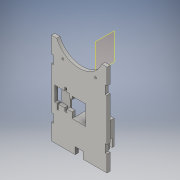
# Autodesk Inventor part: Backhalf
Saved by Autodesk Inventor 2016 (Build 200138000, 138)
## iProperties
Created: 2017-03-04
Part Number: Backhalf
Material: Generic
Document SubType Name: Modeling
Designer: Owner
Density: 1 g/cm^3
Appearance: Default
Author: Owner
Autodesk Inventor part; units mm, degrees
ref_plane "YZ Plane" through (0, 0, 0) normal (1, 0, 0) x (0, 1, 0)
ref_plane "XZ Plane" through (0, 0, 0) normal (0, 1, 0) x (-1, 0, 0)
ref_plane "XY Plane" through (0, 0, 0) normal (0, 0, 1) x (1, 0, 0)
sketch "Sketch1" plane through (0, 0, 0) normal (0, 0, 1) x (1, 0, 0)
  line L0 (31.75, -57.15) -> (31.75, 82.55)
  line L1 (31.75, 82.55) -> (-44.45, 82.55)
  line L2 (-44.45, 82.55) -> (-44.45, -57.15)
  arc A0 (-44.45, -57.15) -> (31.75, -57.15) centre (-6.35, -57.15) ccw
  line L3 (31.75, -57.15) -> (31.75, -209.55)
  line L4 (31.75, -209.55) -> (-44.45, -209.55)
  line L5 (-44.45, -209.55) -> (-44.45, -57.15)
  line L6 (31.75, -57.15) -> (-44.45, -57.15)
  circle A1 centre (-6.35, -57.15) radius 38.1
  point P0 (0, 0)
  dimension "d0" = 152.4
  dimension "d6" = 76.2
  constraints: 14 end point, 3 perpendicular, 2 centre point, 2 point on circle, 2 tangent, 1 coincident, 1 concentric, 1 vertical
  measures "d0" distance of L0.start L3.end
  measures "d6" distance of L3.end L4.end
extrude "Extrusion1" add sketch "Sketch1" against normal blind 5 contours L3 L4 L5 A0
sketch "Sketch2" plane through (0, 0, 0) normal (0, 0, 1) x (1, 0, 0)
  arc A0 (-44.45, -57.15) -> (31.75, -57.15) centre (-6.35, -57.15) ccw projected
  line L0 (31.75, -57.15) -> (31.75, -209.55) projected
  line L1 (-44.45, -57.15) -> (31.75, -57.15)
  line L2 (31.75, -57.15) -> (31.75, -72.15)
  line L3 (31.75, -72.15) -> (-44.45, -72.15)
  line L4 (-44.45, -72.15) -> (-44.45, -57.15)
  point P0 (0, 0)
  dimension "d3" = 15
  constraints: 8 end point, 2 parallel, 1 horizontal, 1 perpendicular, 1 point on line
  measures "d3" distance of L3.end L1.start
extrude "Extrusion2" cut sketch "Sketch2" against normal blind 5 contours L1 A0 L3 | A0 L3 L4 | L0 L3 A0
sketch "Sketch3" plane through (0, 0, -5) normal (0, 0, -1) x (-1, 0, 0)
  line L0 (16.51, -146.85) -> (16.51, -159.55) projected
  line L1 (-3.81, -159.55) -> (-3.81, -146.85) projected
  line L2 (16.51, -159.55) -> (16.51, -161.55)
  line L3 (-3.81, -146.85) -> (-3.81, -144.85)
  line L4 (4.857, -150.5555) -> (16.51, -161.55)
  line L5 (8.3369, -156.3105) -> (-3.81, -144.85)
  line L6 (16.51, -141.135) -> (12.446, -141.135)
  line L7 (16.51, -165.265) -> (12.446, -165.265)
  line L8 (16.51, -141.135) -> (17.51, -141.135)
  line L9 (17.51, -141.135) -> (17.51, -138.135)
  line L10 (17.51, -138.135) -> (-3.81, -138.135)
  line L11 (-3.81, -138.135) -> (-3.81, -163.265)
  line L12 (-3.81, -163.265) -> (-3.81, -164.265)
  line L13 (17.51, -138.135) -> (17.51, -165.265)
  line L14 (17.51, -165.265) -> (17.51, -168.265)
  line L15 (17.51, -168.265) -> (-3.81, -168.265)
  line L16 (-3.81, -168.265) -> (-3.81, -164.265)
  point P0 (0, 0)
  point P1 (17.51, -164.265)
  dimension "d7" = 2
  dimension "d8" = 2
  dimension "d28" = 1
  dimension "d29" = 3
  dimension "d30" = 1
  dimension "d73" = 3
  constraints: 30 end point, 5 perpendicular, 3 horizontal, 3 point on line, 3 vertical, 1 parallel, 4 other
  measures "d7" distance of L0.end L2.end
  measures "d8" distance of L1.end L3.end
  measures "d28" distance of L6.start L8.end
  measures "d29" distance of L8.end L9.end
  measures "d30" distance of L11.end L12.end
  measures "d73" distance of L13.end L14.end
extrude "Extrusion3" cut sketch "Sketch3" against normal blind 5
sketch "Sketch4" plane through (0, 0, -5) normal (0, 0, -1) x (-1, 0, 0)
  line L0 (-31.75, -72.15) -> (-28.673, -72.15) projected
  line L1 (-31.75, -72.15) -> (-36.75, -72.15)
  line L2 (-36.75, -72.15) -> (-36.75, -209.55)
  line L3 (-36.75, -209.55) -> (-36.75, -214.55)
  line L4 (-36.75, -214.55) -> (44.45, -214.55)
  line L5 (44.45, -214.55) -> (49.45, -214.55)
  line L6 (49.45, -214.55) -> (49.45, -72.15)
  line L7 (49.45, -72.15) -> (44.45, -72.15)
  line L8 (44.45, -72.15) -> (44.45, -214.55)
  line L9 (44.45, -214.55) -> (49.45, -214.55)
  line L10 (49.45, -214.55) -> (49.45, -72.15)
  line L11 (49.45, -214.55) -> (-36.75, -214.55)
  line L12 (-36.75, -214.55) -> (-36.75, -209.55)
  line L13 (-36.75, -209.55) -> (49.45, -209.55)
  line L14 (49.45, -209.55) -> (49.45, -214.55)
  line L15 (-36.75, -214.55) -> (-31.75, -214.55)
  line L16 (-31.75, -214.55) -> (-31.75, -72.15)
  line L17 (-31.75, -72.15) -> (-36.75, -72.15)
  line L18 (-36.75, -72.15) -> (-36.75, -214.55)
  point P0 (0, 0)
  dimension "d11" = 5
  dimension "d12" = 5
  dimension "d13" = 5
  constraints: 36 end point, 6 parallel, 6 perpendicular, 4 horizontal, 3 point on line
  measures "d11" distance of L0.start L1.end
  measures "d12" distance of L2.end L3.end
  measures "d13" distance of L4.end L5.end
extrude "Extrusion4" add sketch "Sketch4" against normal blind 5
sketch "Sketch6" plane through (-49.45, -214.55, 0) normal (0, -1, 0) x (1, 0, 0)
  line L0 (32.94, 0) -> (53.26, 0) projected
  line L1 (43.1, 0) -> (36.75, 0)
  line L2 (36.75, 0) -> (49.45, 0)
  line L3 (86.2, -5) -> (0, -5) projected
  line L4 (49.45, 0) -> (36.75, 0)
  line L5 (36.75, 0) -> (36.75, -5)
  line L6 (36.75, -5) -> (49.45, -5)
  line L7 (49.45, -5) -> (49.45, 0)
  point P0 (64.1616, -5)
  dimension "d18" = 6.35
  dimension "d19" = 12.7
  constraints: 12 end point, 2 parallel, 2 point on line, 1 collinear, 1 horizontal, 1 midpoint, 1 perpendicular
  measures "d18" distance of L1.start L1.end
  measures "d19" distance of L1.end L2.end
extrude "Extrusion6" add sketch "Sketch6" along normal blind 10.16
sketch "Sketch7" plane through (0, 0, -5) normal (0, 0, -1) x (-1, 0, 0)
  line L0 (12.7, -224.71) -> (0, -224.71) projected
  line L1 (6.35, -224.71) -> (6.35, -220.9)
  circle A0 centre (6.35, -220.9) radius 1.75
  point P0 (0, 0)
  dimension "d26" = 3.81
  dimension "d27" = 3.5
  constraints: 2 end point, 1 centre point, 1 coincident, 1 midpoint, 1 vertical
  measures "d26" distance of L1.start L1.end
  measures "d27" diameter of A0
extrude "Extrusion7" cut sketch "Sketch7" against normal blind 6.35
sketch "Sketch8" plane through (0, 0, -5) normal (0, 0, -1) x (-1, 0, 0)
  line L0 (44.45, -136.69) -> (28.448, -136.69) projected
  line L1 (44.45, -158.28) -> (44.45, -137.96) projected
  line L2 (44.45, -136.69) -> (44.45, -137.96) projected
  line L3 (44.45, -158.28) -> (44.45, -159.55) projected
  line L4 (44.45, -159.55) -> (28.448, -159.55) projected
  line L5 (39.116, -159.55) -> (40.132, -159.55) projected
  line L6 (39.116, -159.55) -> (39.116, -162.09) projected
  line L7 (40.132, -162.09) -> (39.116, -162.09) projected
  line L8 (40.132, -159.55) -> (40.132, -162.09) projected
  line L9 (25.908, -137.96) -> (21.59, -137.96) projected
  line L10 (21.59, -153.2) -> (21.59, -137.96) projected
  line L11 (21.59, -158.28) -> (21.59, -153.2) projected
  line L12 (25.908, -158.28) -> (21.59, -158.28) projected
  line L13 (25.908, -158.28) -> (25.908, -164.122) projected
  line L14 (25.908, -164.122) -> (28.448, -164.122) projected
  line L15 (28.448, -158.28) -> (28.448, -164.122) projected
  line L16 (44.45, -158.28) -> (28.448, -158.28) projected
  line L17 (44.45, -158.28) -> (44.45, -137.96) projected
  line L18 (44.45, -137.96) -> (28.448, -137.96) projected
  line L19 (28.448, -132.118) -> (28.448, -137.96) projected
  line L20 (25.908, -132.118) -> (28.448, -132.118) projected
  line L21 (25.908, -132.118) -> (25.908, -137.96) projected
  line L22 (25.908, -136.69) -> (21.59, -136.69) projected
  line L23 (21.59, -136.69) -> (21.59, -137.96) projected
  line L24 (25.908, -159.55) -> (21.59, -159.55) projected
  line L25 (21.59, -159.55) -> (16.51, -159.55)
  line L26 (21.59, -146.85) -> (16.51, -146.85)
  line L27 (17.51, -140.135) -> (17.51, -166.265) projected
  line L28 (44.45, -159.55) -> (21.59, -159.55)
  line L29 (21.59, -159.55) -> (21.59, -136.69)
  line L30 (21.59, -136.69) -> (44.45, -136.69)
  line L31 (44.45, -136.69) -> (44.45, -159.55)
  line L32 (28.448, -132.118) -> (25.908, -132.118)
  line L33 (25.908, -132.118) -> (25.908, -136.69)
  line L34 (25.908, -136.69) -> (28.448, -136.69)
  line L35 (28.448, -136.69) -> (28.448, -132.118)
  line L36 (25.908, -159.55) -> (28.448, -159.55)
  line L37 (28.448, -159.55) -> (28.448, -164.122)
  line L38 (28.448, -164.122) -> (25.908, -164.122)
  line L39 (25.908, -164.122) -> (25.908, -159.55)
  line L40 (40.132, -162.09) -> (39.116, -162.09)
  line L41 (39.116, -162.09) -> (39.116, -159.55)
  line L42 (39.116, -159.55) -> (40.132, -159.55)
  line L43 (40.132, -159.55) -> (40.132, -162.09)
  line L44 (16.51, -146.85) -> (21.59, -146.85)
  line L45 (21.59, -146.85) -> (21.59, -159.55)
  line L46 (21.59, -159.55) -> (16.51, -159.55)
  line L47 (16.51, -159.55) -> (16.51, -146.85)
  line L48 (40.132, -159.55) -> (40.64, -159.55)
  line L49 (40.64, -159.55) -> (40.64, -167.805)
  line L50 (40.64, -167.805) -> (39.116, -167.805)
  line L51 (39.116, -167.805) -> (38.608, -167.805)
  line L52 (38.608, -167.805) -> (38.608, -159.55)
  line L53 (40.64, -167.805) -> (38.608, -167.805)
  line L54 (38.608, -167.805) -> (38.608, -159.55)
  line L55 (38.608, -159.55) -> (40.64, -159.55)
  line L56 (40.64, -159.55) -> (40.64, -167.805)
  line L57 (28.448, -136.69) -> (28.948, -136.69)
  line L58 (28.948, -136.69) -> (28.948, -132.118)
  line L59 (28.948, -132.118) -> (28.948, -131.618)
  line L60 (28.948, -131.618) -> (25.908, -131.618)
  line L61 (25.908, -131.618) -> (25.408, -131.618)
  line L62 (25.408, -131.618) -> (25.408, -136.69)
  line L63 (44.45, -148.12) -> (42.0007, -148.12)
  line L64 (28.448, -164.122) -> (28.448, -158.28)
  line L65 (25.908, -164.122) -> (28.448, -164.122)
  line L66 (25.908, -164.122) -> (25.908, -158.28)
  line L67 (28.448, -164.122) -> (25.908, -164.122)
  line L68 (25.908, -164.122) -> (25.908, -159.55)
  line L69 (28.448, -159.55) -> (28.448, -164.122)
  line L70 (28.948, -159.55) -> (28.948, -164.122)
  line L71 (28.948, -164.122) -> (28.948, -164.622)
  line L72 (28.948, -164.622) -> (25.908, -164.622)
  line L73 (25.908, -164.622) -> (25.408, -164.622)
  line L74 (25.408, -164.622) -> (25.408, -159.55)
  line L75 (28.948, -159.55) -> (25.408, -159.55)
  line L76 (25.408, -159.55) -> (25.408, -164.622)
  line L77 (25.408, -164.622) -> (28.948, -164.622)
  line L78 (28.948, -164.622) -> (28.948, -159.55)
  point P0 (0, 0)
  dimension "d33" = 0.508
  dimension "d34" = 8.255
  dimension "d35" = 0.508
  dimension "d45" = 0.5
  dimension "d46" = 0.5
  dimension "d47" = 0.5
  constraints: 100 end point, 14 parallel, 12 perpendicular, 10 horizontal, 9 point on line, 9 symmetric about line, 1 midpoint, 1 vertical, 3 other
  measures "d33" distance of L42.end L48.end
  measures "d34" distance of L48.end L49.end
  measures "d35" distance of L50.end L51.end
  measures "d45" distance of L34.end L57.end
  measures "d46" distance of L58.end L59.end
  measures "d47" distance of L60.end L61.end
extrude "Extrusion8" cut sketch "Sketch8" against normal blind 25.4
ref_plane "Work Plane1" through (-5.588, -193.539, -26.4481) normal (1, 0, 0) x (0, 0, 1)
sketch "Sketch18" plane through (0, 0, -5) normal (0, 0, -1) x (-1, 0, 0)
  line L0 (-36.75, -72.15) -> (-28.673, -72.15) projected
  line L1 (-36.75, -72.15) -> (-36.75, -97.55)
  line L2 (-36.75, -214.55) -> (-36.75, -72.15) projected
  line L3 (-36.75, -97.55) -> (-33.7528, -97.55)
  line L4 (-33.7528, -97.55) -> (-33.7528, -110.25)
  line L5 (-33.7528, -110.25) -> (-36.75, -110.25)
  line L6 (-36.75, -110.25) -> (-36.75, -97.55)
  line L7 (-36.75, -214.55) -> (-36.75, -189.15)
  line L8 (-36.75, -189.15) -> (-33.7528, -189.15)
  line L9 (-33.7528, -189.15) -> (-33.7528, -176.45)
  line L10 (-33.7528, -176.45) -> (-36.75, -176.45)
  line L11 (-36.75, -176.45) -> (-36.75, -189.15)
  line L12 (0, -224.71) -> (12.7, -224.71) projected
  line L13 (6.35, -224.71) -> (6.35, -239.7955)
  line L14 (49.45, -72.15) -> (41.373, -72.15)
  line L15 (49.45, -72.15) -> (49.45, -97.55)
  line L16 (49.45, -214.55) -> (49.45, -72.15)
  line L17 (49.45, -97.55) -> (46.4528, -97.55)
  line L18 (46.4528, -97.55) -> (46.4528, -110.25)
  line L19 (46.4528, -110.25) -> (49.45, -110.25)
  line L20 (49.45, -110.25) -> (49.45, -97.55)
  line L21 (49.45, -214.55) -> (49.45, -189.15)
  line L22 (49.45, -189.15) -> (46.4528, -189.15)
  line L23 (46.4528, -189.15) -> (46.4528, -176.45)
  line L24 (46.4528, -176.45) -> (49.45, -176.45)
  line L25 (49.45, -176.45) -> (49.45, -189.15)
  point P0 (0, 0)
  dimension "d83" = 25.4
  dimension "d84" = 12.7
  dimension "d85" = 2.9972
  dimension "d86" = 25.4
  dimension "d87" = 12.7
  dimension "d88" = 2.9972
  constraints: 46 end point, 11 symmetric about line, 4 parallel, 4 point on line, 2 horizontal, 2 perpendicular, 1 midpoint, 1 vertical
  measures "d83" distance of L0.start L1.end
  measures "d84" distance of L3.end L4.end
  measures "d85" distance of L4.end L5.end
  measures "d86" distance of L2.start L7.end
  measures "d87" distance of L8.end L9.end
  measures "d88" distance of L7.end L8.end
extrude "Extrusion18" cut sketch "Sketch18" against normal blind 10
sketch "Sketch20" plane through (-49.45, -224.71, 0) normal (0, -1, 0) x (1, 0, 0)
  line L0 (36.75, -5) -> (36.75, 0) projected
  line L1 (36.75, -5) -> (49.45, -5)
  line L2 (49.45, -5) -> (49.45, 0)
  line L3 (49.45, 0) -> (36.75, 0)
  line L4 (36.75, 0) -> (36.75, -5)
  constraints: 8 end point, 2 parallel, 1 horizontal, 1 perpendicular
extrude "Extrusion19" cut sketch "Sketch20" against normal blind 20.8946
sketch "Sketch22" plane through (0, 0, -5) normal (0, 0, -1) x (-1, 0, 0)
  line L0 (25.408, -159.55) -> (25.408, -164.622) projected
  line L1 (25.408, -164.622) -> (38.608, -164.622)
  line L2 (38.608, -164.622) -> (38.608, -131.618)
  line L3 (38.608, -131.618) -> (25.408, -131.618)
  line L4 (25.408, -131.618) -> (25.408, -164.622)
  point P0 (0, 0)
  constraints: 8 end point, 2 parallel, 1 horizontal, 1 perpendicular
extrude "Extrusion21" add sketch "Sketch22" along normal blind 2.54
ref_plane "Work Plane2" through (14.732, -52.9, -29.002) normal (1, 0, 0) x (0, 0, -1)
sketch "Sketch24" plane through (14.732, -52.9, -29.002) normal (1, 0, 0) x (0, 0, -1)
  line L0 (0, -25.4) -> (0, -38.1) construction
  line L1 (0, -38.1) -> (3, -38.1) construction
  line L2 (3, 0) -> (3, -38.1) projected
  line L3 (-24.002, 0) -> (3, 0) construction
  line L4 (-24.002, -17.78) -> (-24.002, 0) construction
  line L5 (-5.54, -17.78) -> (-24.002, -17.78) construction
  line L6 (-5.54, -38.1) -> (-5.54, -17.78) construction
  line L7 (-2.54, -38.1) -> (-5.54, -38.1) construction
  line L8 (-2.54, -38.1) -> (-2.54, -25.4) construction
  line L9 (-2.54, -25.4) -> (0, -25.4) construction
  line L10 (-24.002, -115.365) -> (-29.002, -115.365) projected
  line L11 (-24.002, -115.365) -> (-24.002, -133.145)
  line L12 (-24.002, -115.365) -> (2.9982, -115.365)
  line L13 (2.9982, -115.365) -> (2.9982, -153.465)
  line L14 (-24.002, -133.145) -> (-5.5413, -133.145)
  line L15 (-5.5413, -133.145) -> (-5.5413, -153.465)
  line L16 (-5.5413, -153.465) -> (-2.5441, -153.465)
  line L17 (-2.5441, -153.465) -> (-2.5441, -140.765)
  line L18 (-2.5441, -140.765) -> (-0.0041, -140.765)
  line L19 (-0.0041, -140.765) -> (-0.0041, -153.465)
  line L20 (-0.0041, -153.465) -> (2.9982, -153.465)
  point P0 (-29.002, 52.9)
  dimension "d102" = 17.78
  dimension "d103" = 27.0002
  dimension "d104" = 38.1
  dimension "d106" = 18.4607
  dimension "d107" = 20.32
  dimension "d108" = 2.9972
  dimension "d109" = 12.7
  dimension "d110" = 2.54
  constraints: 20 end point, 4 perpendicular, 3 horizontal, 3 vertical
  measures "d102" distance of L10.start L11.end
  measures "d103" distance of L10.start L12.end
  measures "d104" distance of L12.end L13.end
  measures "d106" distance of L11.end L14.end
  measures "d107" distance of L14.end L15.end
  measures "d108" distance of L15.end L16.end
  measures "d109" distance of L16.end L17.end
  measures "d110" distance of L17.end L18.end
extrude "Extrusion23" add sketch "Sketch24" against normal blind 32.04
sketch "Sketch25" plane through (14.732, -206.365, -32.0002) normal (0, 0, -1) x (-1, 0, 0)
  line L0 (27.432, 135.685) -> (27.432, 115.365) projected
  line L1 (4.572, 115.365) -> (4.572, 135.685) projected
  line L2 (27.432, 115.365) -> (32.004, 115.365) projected
  line L3 (0, 0) -> (32.04, 0) projected
  line L4 (32.04, 0) -> (27.468, 0)
  line L5 (0, 0) -> (4.572, 0)
  line L6 (4.572, 0) -> (27.432, 0)
  line L7 (27.432, 0) -> (27.432, 20.32)
  line L8 (27.432, 20.32) -> (4.572, 20.32)
  line L9 (4.572, 20.32) -> (4.572, 0)
  point P0 (14.732, 206.365)
  dimension "d113" = 4.572
  dimension "d114" = 4.572
  dimension "d115" = 20.32
  constraints: 12 end point, 2 parallel, 2 point on line, 1 horizontal, 1 perpendicular
  measures "d113" distance of L3.end L4.end
  measures "d114" distance of L3.start L5.end
  measures "d115" distance of L6.end L7.end
extrude "Extrusion24" cut sketch "Sketch25" against normal blind 10
sketch "Sketch26" plane through (0, 0, -5) normal (0, 0, -1) x (-1, 0, 0)
  circle A0 centre (-19.05, -95.25) radius 2 projected
  circle A1 centre (31.75, -95.25) radius 2 projected
  circle A2 centre (31.75, -95.25) radius 1.5
  circle A3 centre (-19.05, -95.25) radius 1.5
  point P0 (0, 0)
  dimension "d118" = 3
  dimension "d119" = 3
  constraints: 2 centre point, 2 coincident
  measures "d118" diameter of A2
  measures "d119" diameter of A3
extrude "Extrusion25" cut sketch "Sketch26" against normal blind 10 contours A2 | A3
sketch "Sketch27" plane through (14.732, -206.365, -32.0002) normal (0, 0, -1) x (-1, 0, 0)
  line L0 (4.572, 0) -> (4.572, 20.32) projected
  line L1 (4.572, 20.32) -> (27.432, 20.32) projected
  line L2 (27.432, 20.32) -> (27.432, 0) projected
  line L3 (27.432, 0) -> (32.04, 0) projected
  line L4 (32.04, 38.1) -> (32.04, 0) projected
  line L5 (0, 38.1) -> (32.04, 38.1) projected
  line L6 (0, 0) -> (0, 38.1) projected
  line L7 (0, 0) -> (4.572, 0) projected
  point P0 (14.732, 206.365)
extrude "Extrusion26" add sketch "Sketch27" along normal blind 1
sketch "Sketch28" plane through (14.732, -52.9, -29.002) normal (1, 0, 0) x (0, 0, -1)
  line L0 (-2.5441, -140.765) -> (-0.0041, -140.765) projected
  line L1 (-0.0041, -153.465) -> (3.9982, -153.465) projected
  line L2 (-0.0041, -140.765) -> (0.9959, -140.765)
  line L3 (0.9959, -140.765) -> (0.9959, -153.465)
  line L4 (0.9959, -153.465) -> (-0.0041, -153.465)
  line L5 (-0.0041, -153.465) -> (-0.0041, -140.765)
  point P0 (-29.002, 52.9)
  dimension "d124" = 1
  constraints: 8 end point, 2 parallel, 1 horizontal, 1 perpendicular, 1 point on line
  measures "d124" distance between parallel lines of L5 L3
extrude "Extrusion27" cut sketch "Sketch28" against normal blind 3098.8
sketch "Sketch29" plane through (0, 0, -5) normal (0, 0, -1) x (-1, 0, 0)
  line L0 (21.59, -146.85) -> (17.51, -146.85) projected
  line L1 (21.59, -146.85) -> (21.59, -143.04)
  line L2 (21.59, -136.69) -> (21.59, -146.85) projected
  line L3 (21.59, -143.04) -> (17.51, -143.04)
  line L4 (17.51, -143.04) -> (17.51, -146.85)
  line L5 (17.51, -146.85) -> (21.59, -146.85)
  point P0 (0, 0)
  dimension "d127" = 3.81
  constraints: 8 end point, 3 perpendicular, 1 point on line
  measures "d127" distance of L0.start L1.end
extrude "Extrusion28" cut sketch "Sketch29" against normal blind 3098.8
body "Solid1"
